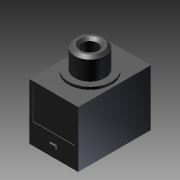
# Autodesk Inventor part: WT_body
Saved by Autodesk Inventor 2011 SP1 (Build 150282100, 282)
## iProperties
Created: 2013-12-24
Part Number: WT_body
Catalog Web Link: www.cadenas.de
Description: WT Body-WT Body
Vendor: NKKSWITCHES
Document SubType Name: Modeling
Designer: PARTuser1
Manufacturer: NKKSWITCHES
Density: 1 g/cm^3
Category: PARTsolutions
Company: NKKSWITCHES
Title: WT_body
Author: Cadenas PARTsolutions
Comments: WT Body
PSOL_IDENT_0: {$CADENAS_DATA\23d-libs\nkkswitches\toggle\wt\parts\wt_body.prj},157 {VTYP=3D},{NB=WT_body},{LINA=WT
PSOL_IDENT_1: _body},{NN=WT Body},{DATE=26.06.2008 07:32:17},{GEOMDATE=26.06.2008 07:32:00},{VERSION=},{LINEID=10}
PSOL_IDENT_2: ,{LINESUBID=-1},{WBVAR=}  {NB=WT_body},{LINA=WT_body},{KT=DUMMY},{PN=WT_body},{D=12.0000}
CNS_NN: WT Body
CNS_NT: WT Body
CNS_NB: WT_body
CNS_NBSYN: $PN.
CNS_LINA: WT_body
CNS_PN: WT_body
CNS_D: 12.0000
SUPPLIER: NKKSWITCHES
ARTICLENO: WT_body
BOMINFO: WT_body
CREATOR: CADENAS GmbH
Autodesk Inventor part; units mm, degrees
sketch "Sketch_1" plane through (0, 0, 0) normal (0, 1, 0) x (-1, 0, 0)
  line L0 (9.7028, 14.4018) -> (-9.7028, 14.4018)
  line L1 (-9.7028, 14.4018) -> (-9.7028, -14.4018)
  line L2 (-9.7028, -14.4018) -> (9.7028, -14.4018)
  line L3 (9.7028, -14.4018) -> (9.7028, 14.4018)
  constraints: 8 end point
extrude "Extrusion1" add sketch "Sketch_1" against normal blind 22.3012
sketch "Sketch_2" plane through (0, 0, 0) normal (0, 1, 0) x (-1, 0, 0)
  circle A0 centre (0, 0) radius 8.5725
  constraints: 1 centre point
extrude "Extrusion2" add sketch "Sketch_2" along normal blind 0.9906
sketch "Sketch_3" plane through (0, 0, 0) normal (1, 0, 0) x (0, 1, 0)
  line L0 (0.9906, 0) -> (9.6012, 0)
  line L1 (9.6012, 0) -> (9.6012, -4.9265)
  line L2 (9.6012, -4.9265) -> (8.5277, -6)
  line L3 (8.5277, -6) -> (0.9906, -6)
  line L4 (0.9906, -6) -> (0.9906, 0)
  line L5 (0.9906, 0) -> (9.6012, 0)
  constraints: 12 end point
revolve "Revolution1" add sketch "Sketch_3" angle 360 about axis through (0, 0.9906, 0) along (0, 1, 0)
sketch "Sketch_10" plane through (0, 0.9906, 0) normal (0, 1, 0) x (1, 0, 0)
  line L0 (-2.9909, 5.2014) -> (2.9909, 5.2014)
  arc A0 (2.9909, 5.2014) -> (-2.9909, 5.2014) centre (0, 0) ccw
  constraints: 2 end point, 2 point on circle, 1 centre point
extrude "Extrusion3" cut sketch "Sketch_10" along normal blind 8.6106
sketch "Sketch5" plane through (0, 9.6012, 0) normal (0, 1, 0) x (1, 0, 0)
  point P0 (0, 0)
hole "Drilling 1" at (0, 9.6012, 0) direction (0, -1, 0) diameter 6 depth 8.6106 countersink diameter 8 countersink angle 90
sketch "Sketch_5" plane through (0, -22.3012, 0) normal (0, 1, 0) x (1, 0, 0)
  line L0 (-8.4328, -13.1318) -> (8.4328, -13.1318)
  line L1 (8.4328, -13.1318) -> (8.4328, 13.1318)
  line L2 (8.4328, 13.1318) -> (-8.4328, 13.1318)
  line L3 (-8.4328, 13.1318) -> (-8.4328, -13.1318)
  constraints: 8 end point
extrude "Extrusion4" cut sketch "Sketch_5" along normal blind 0.254
sketch "Sketch_6" plane through (0, 0, -14.4018) normal (0, 0, 1) x (1, 0, 0)
  line L0 (-8.4328, -1.27) -> (-8.4328, -14.0208)
  line L1 (-8.4328, -14.0208) -> (8.4328, -14.0208)
  line L2 (8.4328, -14.0208) -> (8.4328, -1.27)
  line L3 (8.4328, -1.27) -> (-8.4328, -1.27)
  constraints: 8 end point
extrude "Extrusion5" cut sketch "Sketch_6" along normal blind 0.254
sketch "Sketch_7" plane through (0, 0, 14.4018) normal (0, 0, 1) x (1, 0, 0)
  line L0 (-8.4328, -1.27) -> (-8.4328, -14.0208)
  line L1 (-8.4328, -14.0208) -> (8.4328, -14.0208)
  line L2 (8.4328, -14.0208) -> (8.4328, -1.27)
  line L3 (8.4328, -1.27) -> (-8.4328, -1.27)
  constraints: 8 end point
extrude "Extrusion6" cut sketch "Sketch_7" against normal blind 0.254
sketch "Sketch_8" plane through (0, 0, 0) normal (1, 0, 0) x (0, 1, 0)
  line L0 (-17.3939, 15.113) -> (-18.4034, 15.113)
  line L1 (-18.4034, 15.113) -> (-18.796, 14.4018)
  line L2 (-18.796, 14.4018) -> (-17.3939, 14.4018)
  line L3 (-17.3939, 14.4018) -> (-17.3939, 15.113)
  constraints: 8 end point
extrude "Extrusion7" add sketch "Sketch_8" along normal mid plane 2.54
sketch "Sketch_9" plane through (0, 0, 0) normal (1, 0, 0) x (0, 1, 0)
  line L0 (-17.3939, -14.4018) -> (-18.796, -14.4018)
  line L1 (-18.796, -14.4018) -> (-18.4034, -15.113)
  line L2 (-18.4034, -15.113) -> (-17.3939, -15.113)
  line L3 (-17.3939, -15.113) -> (-17.3939, -14.4018)
  constraints: 8 end point
extrude "Extrusion8" add sketch "Sketch_9" along normal mid plane 2.54
ref_plane "body_to_body2_XY" through (0, -15.2908, 0) normal (0, -1, 0) x (1, 0, 0)
ref_plane "body_to_body2_YZ" through (0, -15.2908, 0) normal (1, 0, 0) x (0, 0, 1)
ref_plane "body_to_body2_ZX" through (0, -15.2908, 0) normal (0, 0, 1) x (0, -1, 0)
ref_plane "body_to_dummy_XY" through (0, 0, 0) normal (0, -1, 0) x (1, 0, 0)
ref_plane "body_to_dummy_YZ" through (0, 0, 0) normal (1, 0, 0) x (0, 0, 1)
ref_plane "body_to_dummy_ZX" through (0, 0, 0) normal (0, 0, 1) x (0, -1, 0)
ref_plane "body_to_terminal_XY" through (0, -22.3012, 0) normal (0, 1, 0) x (1, 0, 0)
ref_plane "body_to_terminal_YZ" through (0, -22.3012, 0) normal (1, 0, 0) x (0, 0, -1)
ref_plane "body_to_terminal_ZX" through (0, -22.3012, 0) normal (0, 0, -1) x (0, 1, 0)
ref_plane "body_to_toggle_XY" through (0, 2.4003, 0) normal (0, -1, 0) x (1, 0, 0)
ref_plane "body_to_toggle_YZ" through (0, 2.4003, 0) normal (1, 0, 0) x (0, 0, 1)
ref_plane "body_to_toggle_ZX" through (0, 2.4003, 0) normal (0, 0, 1) x (0, -1, 0)
ref_plane "body_to_washer_XY" through (0, 0.9906, 0) normal (0, -1, 0) x (1, 0, 0)
ref_plane "body_to_washer_YZ" through (0, 0.9906, 0) normal (1, 0, 0) x (0, 0, 1)
ref_plane "body_to_washer_ZX" through (0, 0.9906, 0) normal (0, 0, 1) x (0, -1, 0)
body "Solid1"
